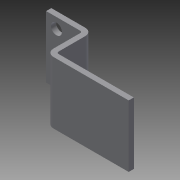
# Autodesk Inventor part: Encoder Mount 2
Saved by Autodesk Inventor 2013 (Build 170138000, 138)
## iProperties
Created: 2013-02-02
Part Number: Encoder Mount 2
Material: Generic
Document SubType Name: Sheet Metal
Designer: actoennies
Density: 1 g/cm^3
Sheet Metal Rule: Default
Author: actoennies
Autodesk Inventor part; units mm, degrees
ref_plane "YZ Plane" through (0, 0, 0) normal (1, 0, 0) x (0, 1, 0)
ref_plane "XZ Plane" through (0, 0, 0) normal (0, 1, 0) x (-1, 0, 0)
ref_plane "XY Plane" through (0, 0, 0) normal (0, 0, 1) x (1, 0, 0)
sketch "Sketch1" plane through (0, 0, 0) normal (0, 0, 1) x (1, 0, 0)
  line L0 (0, 0) -> (0, 38.1)
  line L1 (0, 38.1) -> (19.05, 38.1)
  line L2 (19.05, 38.1) -> (19.05, 0)
  line L3 (19.05, 0) -> (0, 0)
  circle A0 centre (6.35, 31.75) radius 3.3782
  circle A1 centre (6.35, 6.35) radius 3.3782
  dimension "d0" = 38.1
  dimension "d1" = 19.05
  dimension "d2" = 6.7564
  dimension "d3" = 6.7564
  dimension "d4" = 25.4
  dimension "d5" = 6.35
  dimension "d6" = 6.35
  dimension "d7" = 6.35
  measures "d0" distance of L0.start L0.end
  measures "d1" distance of L0.end L1.end
  measures "d2" diameter of A0
  measures "d3" diameter of A1
  measures "d4" distance of A1.centre A0.centre
  measures "d5" distance from line of L1 A0.centre
  measures "d6" distance from line of L0 A0.centre
  measures "d7" distance from line of L0 A1.centre
extrude "Plate1" add sketch "Sketch1" along normal blind 3.175
sketch "Sketch2" plane through (15.875, 38.1, 0) normal (1, 0, 0) x (0, 1, 0)
  line L0 (-38.1, 0) -> (0, 0)
  line L1 (0, 0) -> (0, 50.8)
  line L2 (0, 50.8) -> (-38.1, 50.8)
  line L3 (-38.1, 50.8) -> (-38.1, 0)
  constraints: 6 end point, 1 horizontal, 1 perpendicular, 1 vertical
edge flange "Flange1" height 50.8 angle 90 thickness 3.175 bend radius 1.27 thickness toward (1, 0, 0) relief straight relief width 3.175 relief depth 1.5875 edges at (19.05, 19.05, 3.175) wall of the first edge with corners at (15.875, 0, 0) (15.875, 38.1, 0) (15.875, 38.1, 50.8) (15.875, 0, 50.8)
bend "Bend1"
corner "Corner1"
sketch "Sketch3" plane through (15.875, 0, 47.625) normal (0, 0, 1) x (1, 0, 0)
  line L0 (0, 38.1) -> (0, 0)
  line L1 (0, 0) -> (57.15, 0)
  line L2 (57.15, 0) -> (57.15, 38.1)
  line L3 (57.15, 38.1) -> (0, 38.1)
  constraints: 6 end point, 1 horizontal, 1 perpendicular, 1 vertical
edge flange "Flange2" height 57.15 angle 90 thickness 3.175 bend radius 1.27 thickness toward (0, 0, 1) relief straight relief width 3.175 relief depth 1.5875 edges at (19.05, 19.05, 50.8) wall of the first edge with corners at (15.875, 38.1, 47.625) (15.875, 0, 47.625) (73.025, 0, 47.625) (73.025, 38.1, 47.625)
bend "Bend2"
corner "Corner2"
sketch "Sketch4" plane through (73.025, 0, 50.8) normal (0, 0, 1) x (1, 0, 0)
  arc A0 (-25.9444, 20.5217) -> (-24.767, 22.1384) centre (-22.225, 19.05) ccw projected
  line L0 (-24.767, 22.1384) -> (-24.0613, 21.6245) projected
  line L1 (-24.0613, 21.6245) -> (-25.2388, 20.0078) projected
  line L2 (-25.2388, 20.0078) -> (-25.9444, 20.5217) projected
  circle A1 centre (-22.225, 19.05) radius 6.35
  point P0 (-73.025, 0)
  dimension "d29" = 12.7
  constraints: 1 centre point, 1 coincident
  measures "d29" diameter of A1
extrude "Cut1" cut sketch "Sketch4" against normal blind 3.175 contours L2 L1 L0 A0 | A1
sketch "Sketch5" plane through (73.025, 0, 50.8) normal (0, 0, 1) x (1, 0, 0)
  circle A0 centre (-5.969, 19.05) radius 1.4351 projected
  circle A1 centre (-45.2374, 19.05) radius 1.4351 projected
  circle A2 centre (-38.481, 19.05) radius 1.4351 projected
  point P0 (-73.025, 0)
extrude "Cut2" cut sketch "Sketch5" against normal blind 3.175
equation "\"d31\" = Thickness"
equation "\"d33\" = Thickness"
equation "\"d9\" = BendReliefWidth"
equation "\"d10\" = BendReliefDepth"
equation "\"d11\" = MinimumRemnant"
equation "\"d12\" = BendRadius"
equation "\"d16\" = CornerReliefSize"
equation "\"d17\" = GapSize"
equation "\"d18\" = JacobiRadiusSize"
equation "\"d19\" = BendReliefWidth"
equation "\"d20\" = BendReliefDepth"
equation "\"d21\" = MinimumRemnant"
equation "\"d22\" = BendRadius"
equation "\"d26\" = CornerReliefSize"
equation "\"d27\" = GapSize"
equation "\"d28\" = JacobiRadiusSize"
equation "\"BendRadius\" = Thickness"
equation "\"BendReliefWidth\" = Thickness"
equation "\"BendReliefDepth\" = 0.5 * Thickness"
equation "\"CornerReliefSize\" = 4 * Thickness"
equation "\"MinimumRemnant\" = 2 * Thickness"
equation "\"TransitionRadius\" = BendRadius"
equation "\"JacobiRadiusSize\" = BendRadius"
equation "\"GapSize\" = Thickness"
equation "\"d8\" = BendRadius"
equation "\"Thickness\" = 3.175"
body "Solid1"
